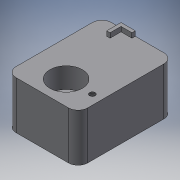
# Autodesk Inventor part: ChipHolder
Saved by Autodesk Inventor 2019 (Build 230136000, 136)
## iProperties
Created: 2019-08-13
Part Number: ChipHolder
Material: Generic
Document SubType Name: Modeling
Designer: aorfi
Density: 1 g/cm^3
Appearance: Default
Author: aorfi
Autodesk Inventor part; units mm, degrees
ref_plane "YZ Plane" through (0, 0, 0) normal (1, 0, 0) x (0, 1, 0)
ref_plane "XZ Plane" through (0, 0, 0) normal (0, 1, 0) x (-1, 0, 0)
ref_plane "XY Plane" through (0, 0, 0) normal (0, 0, 1) x (1, 0, 0)
sketch "Sketch1" plane through (0, 0, 0) normal (0, 1, 0) x (-1, 0, 0)
  line L0 (-7.5, 10) -> (7.5, 10)
  line L1 (7.5, 10) -> (7.5, -10)
  line L2 (7.5, -10) -> (-7.5, -10)
  line L3 (-7.5, -10) -> (-7.5, 10)
  line L4 (-7.5, 10) -> (7.5, -10) construction
  line L5 (7.5, 10) -> (-7.5, -10) construction
  point P0 (0, 0)
  dimension "d0" = 15
  dimension "d1" = 20
  constraints: 12 end point, 2 midpoint, 2 parallel, 1 horizontal, 1 perpendicular
  measures "d0" distance of L1.end L2.end
  measures "d1" distance of L0.end L1.end
extrude "Extrusion1" add sketch "Sketch1" along normal mid plane 10
sketch "Sketch2" plane through (0, 5, 0) normal (0, 1, 0) x (1, 0, 0)
  line L0 (-3.5, 7) -> (-3.5, 10)
  line L1 (-3.5, 10) -> (-0.5, 10)
  line L2 (-0.5, 10) -> (-0.5, 9.3)
  line L3 (-0.5, 9.3) -> (-2.8, 9.3)
  line L4 (-2.8, 9.3) -> (-2.8, 7)
  line L5 (-2.8, 7) -> (-3.5, 7)
  line L6 (7.5, 10) -> (-7.5, 10) projected
  line L7 (-7.5, 10) -> (-7.5, -10) projected
  point P0 (0, 0)
  dimension "d4" = 3
  dimension "d5" = 0.7
  dimension "d7" = 4
  constraints: 12 end point, 4 perpendicular, 2 horizontal, 2 vertical, 1 collinear
  measures "d4" distance of L0.start L0.end
  measures "d5" distance of L4.end L0.start
  measures "d7" distance between parallel lines of L7 L0
extrude "Extrusion2" add sketch "Sketch2" along normal blind 1
fillet "Fillet1" radius 2 4 edges at (-7.5, 0, -10) (-7.5, 0, 10) (7.5, 0, 10) (7.5, 0, -10)
sketch "Sketch4" plane through (0, 5, 0) normal (0, 1, 0) x (1, 0, 0)
  line L0 (7.5, -8) -> (7.5, 8) projected
  line L1 (5.5, 10) -> (-0.5, 10) projected
  line L2 (-7.5, 8) -> (-7.5, -8) projected
  point P0 (0, 0)
  point P1 (5.5, 4)
  point P2 (-5.5, 4)
  dimension "d19" = 2
  dimension "d29" = 6
  dimension "d49" = 2
  constraints: 1 horizontal alignment
  measures "d19" distance from line of L0 point (5.5, 4)
  measures "d29" distance from line of L1 point (5.5, 4)
  measures "d49" distance from line of L2 point (-5.5, 4)
hole "Hole2" at (5.5, 5, -4) at (-5.5, 5, -4) direction (0, -1, 0) diameter 1.181 end through all thread size "0-80 UNF" class "2B" standard "ANSI Unified Screw Threads"
sketch "Sketch6" plane through (0, -5, 0) normal (0, -1, 0) x (1, 0, 0)
  line L0 (5.5, 10) -> (-5.5, 10) projected
  point P0 (0, 0)
  point P1 (0, 5)
  dimension "d38" = 5
  constraints: 1 vertical alignment
  measures "d38" distance from line of L0 point (0, 5)
hole "Hole4" at (0, -5, 5) direction (0, 1, 0) diameter 4.496 end through all clearance for "Flat Head Machine Screw (82)" size "#8" standard "Ansi Unified Screw Threads"
sketch "Sketch7" plane through (0, 5, 0) normal (0, 1, 0) x (1, 0, 0)
  circle A0 centre (0, -5) radius 2.248 projected
  circle A1 centre (0, -5) radius 3.4
  point P0 (0, 0)
  dimension "d46" = 6.8
  constraints: 1 centre point, 1 coincident
  measures "d46" diameter of A1
extrude "Extrusion3" cut sketch "Sketch7" against normal blind 4.3
equation "\"d49\" = d19"
body "Solid1"
